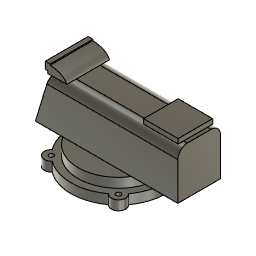
Base (Autodesk Fusion 360 design; units mm, degrees)
Autodesk Fusion 360 part; units mm, degrees
sketch "Sketch1" plane through (0, 0, 0) normal (0, 0, 1) x (1, 0, 0)
  circle A0 centre (0, 0) radius 127
  circle A1 centre (89.8026, 89.8026) radius 19.05
  line L0 (0, 0) -> (112.832, 112.832) construction
  line L1 (0, 0) -> (102.3264, 0) construction
  line L2 (86.9867, 108.6433) -> (69.83, 106.0791)
  line L3 (108.6433, 86.9867) -> (106.0791, 69.83)
  line L4 (-86.9867, 108.6433) -> (-69.83, 106.0791)
  circle A2 centre (-89.8026, 89.8026) radius 19.05
  line L5 (-108.6433, 86.9867) -> (-106.0791, 69.83)
  line L6 (-108.6433, -86.9867) -> (-106.0791, -69.83)
  circle A3 centre (-89.8026, -89.8026) radius 19.05
  line L7 (-86.9867, -108.6433) -> (-69.83, -106.0791)
  line L8 (86.9867, -108.6433) -> (69.83, -106.0791)
  circle A4 centre (89.8026, -89.8026) radius 19.05
  line L9 (108.6433, -86.9867) -> (106.0791, -69.83)
  dimension "d1" = 254
  dimension "d2" = 38.1
  dimension "d3" = 45
  dimension "d7" = 360
  constraint coincident A0.centre L0.start
  constraint coincident A0 A1.centre
  constraint horizontal L1
  constraint coincident A1 L2.start
  constraint coincident A0 L2.end
  constraint coincident A1.centre L0
  constraint tangent A1 L2
  constraint symmetric L0 L2.start L3.start
  constraint symmetric L0 L2.end L3.end
  measures "d1" diameter of A0
  measures "d2" diameter of A1
  measures "d3" angle of L0 L1
extrude "Extrude1" add sketch "Sketch1" along normal blind 25.4 contours A0 A1 A2 A3 A4 | A0 A1 | A0 A1 | A0 A4 | A0 A4 | A0 A2 | A0 A2 | A0 A3 | A0 A3
sketch "Sketch2" plane through (0, 0, 25.4) normal (0, 0, 1) x (-1, 0, 0)
  arc A0 (-75.3598, 102.2247) -> (-102.2247, 75.3598) centre (-89.8026, 89.8026) ccw
  arc A1 (-102.2247, 75.3598) -> (-102.2247, -75.3598) centre (0, 0) ccw
  arc A2 (-102.2247, -75.3598) -> (-75.3598, -102.2247) centre (-89.8026, -89.8026) ccw
  arc A3 (-75.3598, -102.2247) -> (75.3598, -102.2247) centre (0, 0) ccw
  arc A4 (75.3598, -102.2247) -> (102.2247, -75.3598) centre (89.8026, -89.8026) ccw
  arc A5 (102.2247, -75.3598) -> (102.2247, 75.3598) centre (0, 0) ccw
  arc A6 (102.2247, 75.3598) -> (75.3598, 102.2247) centre (89.8026, 89.8026) ccw
  arc A7 (75.3598, 102.2247) -> (-75.3598, 102.2247) centre (0, 0) ccw
  circle A8 centre (89.8026, -89.8026) radius 6.35
  circle A9 centre (89.8026, 89.8026) radius 6.35
  circle A10 centre (-89.8026, 89.8026) radius 6.35
  circle A11 centre (-89.8026, -89.8026) radius 6.35
  dimension "d10" = 12.7
  dimension "d12" = 360
  constraint concentric A4 A8
  measures "d10" diameter of A8
extrude "Extrude2" cut sketch "Sketch2" against normal through all contours A8 | A9 | A10 | A11
sketch "Sketch3" plane through (0, 0, 25.4) normal (0, 0, 1) x (-1, 0, 0)
  circle A0 centre (89.8026, 89.8026) radius 6.35
  circle A1 centre (-89.8026, 89.8026) radius 6.35
  circle A2 centre (89.8026, -89.8026) radius 6.35
  circle A3 centre (-89.8026, -89.8026) radius 6.35
  arc A4 (-75.3598, 102.2247) -> (-102.2247, 75.3598) centre (-89.8026, 89.8026) ccw
  arc A5 (-102.2247, 75.3598) -> (-102.2247, -75.3598) centre (0, 0) ccw
  arc A6 (-102.2247, -75.3598) -> (-75.3598, -102.2247) centre (-89.8026, -89.8026) ccw
  arc A7 (-75.3598, -102.2247) -> (75.3598, -102.2247) centre (0, 0) ccw
  arc A8 (75.3598, -102.2247) -> (102.2247, -75.3598) centre (89.8026, -89.8026) ccw
  arc A9 (102.2247, -75.3598) -> (102.2247, 75.3598) centre (0, 0) ccw
  arc A10 (102.2247, 75.3598) -> (75.3598, 102.2247) centre (89.8026, 89.8026) ccw
  arc A11 (75.3598, 102.2247) -> (-75.3598, 102.2247) centre (0, 0) ccw
  circle A12 centre (0, 0) radius 107.95
  dimension "d14" = 215.9
  constraint coincident A5.centre A7.centre
  measures "d14" diameter of A12
extrude "Extrude3" add sketch "Sketch3" along normal blind 25.4 contours A12
sketch "Sketch4" plane through (0, 0, 50.8) normal (0, 0, 1) x (-1, 0, 0)
  circle A0 centre (0, 0) radius 107.95
  line L0 (165.1, -57.15) -> (-215.9, -57.15)
  line L1 (-215.9, -57.15) -> (-215.9, 57.15)
  line L2 (-215.9, 57.15) -> (165.1, 57.15)
  line L3 (165.1, 57.15) -> (165.1, -57.15)
  dimension "d17" = 57.15
  dimension "d18" = 114.3
  dimension "d20" = 381
  dimension "d60" = 165.1
  constraint horizontal L0
  constraint vertical L1
  constraint horizontal L2
  constraint vertical L3
  measures "d17" distance of A0.centre L2
  measures "d18" distance of L0.end L1.end
  measures "d20" distance of L0.start L0.end
  measures "d60" distance of A0.centre L3
extrude "Extrude4" add sketch "Sketch4" along normal blind 127 contours A0 L0 L2 | A0 L0 L2 L3 | A0 L0 L1 L2
shell "Shell2" thickness 19.05 removed faces 1 at (-165.1, 19.05, 135.4667)
chamfer "Chamfer1" distance 38.1 distance2 127 1 edges at (-165.1, 0, 177.8) measured on face at (-38.1, 19.05, 177.8)
sketch "Sketch5" plane through (0, 57.15, 0) normal (0, 1, 0) x (-1, 0, 0)
  line L0 (165.1, 50.8) -> (127, 177.8)
  line L1 (127, 177.8) -> (-215.9, 177.8)
  line L2 (-215.9, 177.8) -> (-215.9, 50.8)
  line L3 (-215.9, 50.8) -> (-91.581, 50.8)
  line L4 (-91.581, 50.8) -> (91.581, 50.8)
  line L5 (91.581, 50.8) -> (165.1, 50.8)
  line L6 (132.08, 177.8) -> (81.28, 177.8)
  spline S0 degree 5 poles (81.28, 177.8) (81.7967, 178.9642) (82.9768, 181.2609) (85.1865, 184.611) (89.0734, 188.8745) (96.2665, 193.6995) (105.0653, 196.9016) (114.237, 198.7472) (121.6777, 199.6911) (125.73, 200.0913) knots 0 0 0 0 0 0 0.2 0.4 0.6 0.8 1 1 1 1 1 1
  line L7 (114.5582, 198.9879) -> (136.9018, 201.1946)
  line L8 (125.73, 200.0913) -> (125.73, 184.15)
  line L9 (125.73, 184.15) -> (132.08, 184.15)
  line L10 (132.08, 184.15) -> (132.08, 177.8)
  point P0 (127, 177.8)
  dimension "d27" = 50.8
  dimension "d33" = 6.35
  dimension "d56" = 6.35
  dimension "d57" = 15.9413
  dimension "d64" = 5.08
  constraint midpoint S0.end L7
  constraint perpendicular L8 L9
  constraint perpendicular L6 L10
  constraint coincident L1 L6.end
  constraint perpendicular L9 L10
  constraint collinear L1 L6
  measures "d27" distance of L6.start L6.end
  measures "d33" distance of L8.end L9.end
  measures "d56" distance of L6.start L9.end
  measures "d57" distance of S0.end L8.end
  measures "d64" distance of L10 P0
fillet "Fillet1" radius 25.4 1 edges at (44.45, -57.15, 177.8)
fillet "Fillet1" radius 25.4 1 edges at (44.45, 57.15, 177.8)
extrude "Extrude5" add sketch "Sketch5" against normal up to surface (114.3 mm away) contours L1 L6 S0 L8 L9 L10
sketch "Sketch7" plane through (-125.73, 0, 0) normal (-1, 0, 0) x (0, -1, 0)
  line L0 (57.15, 184.15) -> (57.15, 200.0913)
  line L1 (57.15, 200.0913) -> (-57.15, 200.0913)
  line L2 (-57.15, 200.0913) -> (-57.15, 184.15)
  line L3 (-57.15, 184.15) -> (57.15, 184.15)
  line L4 (-57.15, 184.15) -> (57.15, 184.15)
  line L5 (57.15, 184.15) -> (57.15, 203.2)
  line L6 (57.15, 203.2) -> (-57.15, 203.2)
  line L7 (-57.15, 203.2) -> (-57.15, 184.15)
  dimension "d34" = 19.05
  constraint horizontal L4
  constraint vertical L5
  constraint horizontal L6
  constraint vertical L7
  constraint coincident L2.end L3.start
  constraint collinear L0 L5
  measures "d34" distance of L2.end L6.end
extrude "Extrude7" add sketch "Sketch7" along normal blind 12.7
sketch "Sketch10" plane through (0, 0, 19.05) normal (0, 0, 1) x (-1, 0, 0)
  circle A0 centre (0, 0) radius 88.9
  line L0 (-38.1, -15.875) -> (38.1, -15.875)
  line L1 (38.1, -15.875) -> (38.1, 15.875)
  line L2 (38.1, 15.875) -> (-38.1, 15.875)
  line L3 (-38.1, 15.875) -> (-38.1, -15.875)
  line L4 (-38.1, -15.875) -> (38.1, 15.875) construction
  line L5 (38.1, -15.875) -> (-38.1, 15.875) construction
  dimension "d43" = 76.2
  dimension "d44" = 31.75
  constraint horizontal L0
  constraint perpendicular L0 L1
  constraint parallel L0 L2
  constraint parallel L1 L3
  constraint coincident L4 A0.centre
  constraint coincident L5 A0.centre
  constraint coincident A0.centre origin
  measures "d43" distance of L1.end L2.end
  measures "d44" distance of L0.end L1.end
ref_plane "WorkPlane1" through (-38.1, 0, 19.05) normal (-1, 0, 0) x (0, -1, 0)
sketch "Sketch11" plane through (-38.1, 0, 19.05) normal (-1, 0, 0) x (0, 1, 0)
extrude "Extrude9" add sketch "Sketch10" along normal blind 101.6 contours L0 L1 L2 L3
sketch "Sketch12" plane through (-38.1, 0, 0) normal (-1, 0, 0) x (0, -1, 0)
  line L0 (-15.875, 19.05) -> (15.875, 19.05)
  line L1 (15.875, 19.05) -> (15.875, 120.65)
  line L2 (15.875, 120.65) -> (-15.875, 120.65)
  line L3 (-15.875, 120.65) -> (-15.875, 19.05)
  line L4 (0, 120.65) -> (0.0466, 72.8751) construction
  line L5 (-15.875, 96.3922) -> (15.875, 96.3922) construction
  circle A0 centre (0, 96.3922) radius 12.7
  dimension "d51" = 25.4
  constraint midpoint L2 L4.start
  constraint coincident L3 L5.start
  constraint coincident L1 L5.end
  constraint perpendicular L1 L5
  constraint midpoint L5 A0.centre
  measures "d51" diameter of A0
extrude "Extrude10" cut sketch "Sketch12" against normal blind 76.2 contours A0
thread "Thread2" "ANSI Unified Screw Threads 1.0 1-8 UNC 3B" major diameter 25.4 minor diameter 22.159 pitch 3.175 angle 60 resizes the face on face at (12.7, -12.6842, 95.7592)
sketch "Sketch13" plane through (0, 0, 177.8) normal (0, 0, 1) x (-1, 0, 0)
  line L0 (81.28, 31.75) -> (-215.9, 31.75)
  line L1 (-215.9, 31.75) -> (-215.9, -31.75)
  line L2 (-215.9, -31.75) -> (81.28, -31.75)
  line L3 (-206.0564, -46.0136) -> (-113.6358, -46.0136)
  line L4 (-113.6358, -46.0136) -> (-113.6358, 46.4069)
  line L5 (-113.6358, 46.4069) -> (-206.0564, 46.4069)
  line L6 (-206.0564, 46.4069) -> (-206.0564, -46.0136)
  line L7 (-206.0564, -46.0136) -> (-113.6358, 46.4069) construction
  line L8 (-113.6358, -46.0136) -> (-206.0564, 46.4069) construction
  line L9 (12.7, 0.1966) -> (-226.06, 0.1966) construction
  line L10 (81.28, -31.75) -> (81.28, 31.75)
  point P0 (-159.8461, 0.1966)
  constraint horizontal L3
  constraint perpendicular L3 L4
  constraint parallel L3 L5
  constraint parallel L4 L6
  constraint coincident L7 P0
  constraint coincident L8 P0
  constraint perpendicular L1 L9
  constraint midpoint L7 P0
  constraint equal L3 L6
  constraint coincident P0 L9
extrude "Extrude11" add sketch "Sketch13" along normal blind 12.7 contours L0 L2 L4 L6 | L0 L4 L5 L6 | L2 L3 L4 L6
equation "d18 = ( 2.25 * 2 ) * 1 in"
